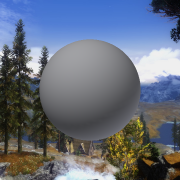
# Autodesk Inventor part: Boulder
Saved by Autodesk Inventor 2015 SP1 (Build 190203100, 203)
## iProperties
Created: 2016-01-20
Part Number: Boulder
Material: Generic
Document SubType Name: Modeling
Designer: TheeTimatahee
Density: 1 g/cm^3
Appearance: Default
Mass: 8580.25 g
Surface Area: 2026.83 cm^2
Volume: 8580.25 cm^3
Author: TheeTimatahee
Autodesk Inventor part; units mm, degrees
ref_plane "YZ Plane" through (0, 0, 0) normal (1, 0, 0) x (0, 1, 0)
ref_plane "XZ Plane" through (0, 0, 0) normal (0, 1, 0) x (-1, 0, 0)
ref_plane "XY Plane" through (0, 0, 0) normal (0, 0, 1) x (1, 0, 0)
sketch "Sketch1" plane through (0, 0, 0) normal (0, 0, 1) x (1, 0, 0)
  circle A0 centre (0, 0) radius 127
  line L0 (0, 127) -> (0, -127)
  dimension "d0" = 254
  constraints: 2 end point, 2 point on circle, 1 centre point, 1 coincident, 1 vertical
  measures "d0" diameter of A0
revolve "Revolution1" add sketch "Sketch1" angle 360 about axis through (0, 127, 0) along (0, -1, 0) picked at (-39.5824, 15.0116) contours L0 A0
body "Solid1"
